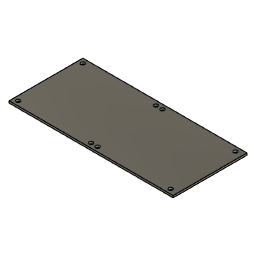
Color Clock asssebly v13 (Autodesk Fusion 360 archive; units mm, degrees)
design "prototype board test"
Autodesk Fusion 360 part; units mm, degrees
sketch "Sketch1" plane through (0, 0, 0) normal (0, 0, 1) x (1, 0, 0)
  line L0 (0, 0) -> (50, 0)
  line L1 (50, 0) -> (50, 45)
  line L2 (50, 45) -> (0, 45)
  line L3 (0, 45) -> (0, 0)
  line L4 (47.25, 42.25) -> (2.75, 42.25)
  line L5 (2.75, 42.25) -> (2.75, 2.75)
  line L6 (2.75, 2.75) -> (47.25, 2.75)
  line L7 (47.25, 2.75) -> (47.25, 42.25)
  line L8 (47.25, 42.25) -> (2.75, 2.75) construction
  line L9 (2.75, 42.25) -> (47.25, 2.75) construction
  line L10 (50, 45) -> (0, 0) construction
  circle A0 centre (2.75, 42.25) radius 1.2
  circle A1 centre (2.75, 2.75) radius 1.2
  circle A2 centre (47.25, 42.25) radius 1.2
  circle A3 centre (47.25, 2.75) radius 1.2
  line L11 (95.75, 2.75) -> (95.75, 42.25)
  line L12 (51.25, 2.75) -> (95.75, 2.75)
  line L13 (98.5, 45) -> (48.5, 0) construction
  line L14 (51.25, 42.25) -> (95.75, 2.75) construction
  line L15 (95.75, 42.25) -> (51.25, 2.75) construction
  circle A4 centre (51.25, 42.25) radius 1.2
  circle A5 centre (51.25, 2.75) radius 1.2
  line L16 (95.75, 42.25) -> (51.25, 42.25)
  circle A6 centre (95.75, 42.25) radius 1.2
  circle A7 centre (95.75, 2.75) radius 1.2
  line L17 (51.25, 42.25) -> (51.25, 2.75)
  line L18 (50, 45) -> (100, 45)
  line L19 (100, 45) -> (100, 0)
  line L20 (100, 0) -> (50, 0)
  line L21 (50, 0) -> (50, 45)
  point P0 (25, 22.5)
  point P1 (73.5, 22.5)
  dimension "d1" = 50
  dimension "d2" = 44.5
  dimension "d3" = 39.5
  dimension "d4" = 2.4
  dimension "d5" = 2.4
  dimension "d6" = 2.4
  dimension "d7" = 2.4
  dimension "d12" = 45
  dimension "d14" = 44.5
  dimension "d15" = 39.5
  dimension "d16" = 2.4
  dimension "d17" = 2.4
  dimension "d18" = 2.4
  dimension "d19" = 2.4
  dimension "d22" = 4
  dimension "d23" = 100
  dimension "d24" = 45
  dimension "d25" = 4.25
  constraint horizontal L0
  constraint vertical L1
  constraint horizontal L2
  constraint vertical L3
  constraint coincident L0.start L3.end
  constraint horizontal L4
  constraint perpendicular L4 L5
  constraint parallel L4 L6
  constraint parallel L5 L7
  constraint coincident L8 P0
  constraint coincident L9 P0
  constraint midpoint P0 L10
  constraint coincident L4.end L5.start
  constraint coincident L5.end L6.start
  constraint coincident L4.start L7.end
  constraint coincident L6.end L7.start
  constraint horizontal L16
  constraint perpendicular L16 L17
  constraint parallel L12 L16
  constraint parallel L11 L17
  constraint coincident P1 L15
  constraint coincident P1 L14
  constraint midpoint P1 L13
  constraint coincident L14.start A4.centre
  constraint coincident L12.start L15.end
  constraint coincident L11.end L15.start
  constraint coincident L11.start L12.end
  constraint horizontal L18
  constraint vertical L19
  constraint horizontal L20
  constraint vertical L21
  measures "d1" distance of L0.start L0.end
  measures "d2" distance of L5.end L6.end
  measures "d3" distance of L4.end L5.end
  measures "d4" diameter of A0
  measures "d5" diameter of A1
  measures "d6" diameter of A2
  measures "d7" diameter of A3
  measures "d12" distance of L0 L2
  measures "d14" distance of L11.start L12.start
  measures "d15" distance of L14.start L12.start
  measures "d16" diameter of A4
  measures "d17" diameter of A5
  measures "d18" diameter of A6
  measures "d19" diameter of A7
  measures "d22" distance of L4.start L14.start
  measures "d23" distance of L3 L19
  measures "d24" distance of L18 L20
  measures "d25" distance of L11 L19
extrude "Extrude1" add sketch "Sketch1" along normal blind 1.2 contours L0 L1 L2 L3 L21 | L4 L5 L6 L7 A0 A1 A2 A3
extrude "Extrude3" add sketch "Sketch1" along normal blind 1.2 contours L1 L18 L19 L20 L21 | L11 L12 A4 A5 L16 A6 A7 L17

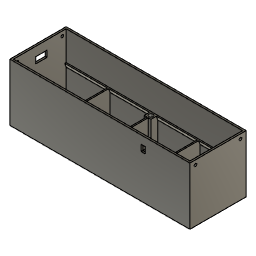
design "Shell"
Autodesk Fusion 360 part; units mm, degrees
derive "DerivedContext1" from "Color Clock asssebly v3"
derive "DerivedContext2" from "Color Clock asssebly v10"
sketch "Sketch1" plane through (0, 0, 0) normal (0, 0, 1) x (1, 0, 0)
  line L0 (0, 0) -> (160, 0)
  line L1 (160, 0) -> (160, 40)
  line L2 (160, 40) -> (0, 40)
  line L3 (0, 40) -> (0, 0)
  dimension "d1" = 160
  dimension "d2" = 40
  constraint horizontal L0
  constraint vertical L1
  constraint horizontal L2
  constraint vertical L3
  constraint coincident L0.start L3.end
  measures "d1" distance of L0.start L0.end
  measures "d2" distance of L0.start L2.end
extrude "Extrude1" add sketch "Sketch1" along normal blind 3 makes body 1
sketch "Sketch2" plane through (0, 0, 3) normal (0, 0, 1) x (-1, 0, 0)
  line L0 (0, -40) -> (0, 0)
  line L1 (0, 0) -> (-160, 0)
  line L2 (-160, 0) -> (-160, -40)
  line L3 (-160, -40) -> (0, -40)
  line L4 (-1.6, -1.6) -> (-158.4, -1.6)
  line L5 (-158.4, -1.6) -> (-158.4, -38.4)
  line L6 (-158.4, -38.4) -> (-1.6, -38.4)
  line L7 (-1.6, -38.4) -> (-1.6, -1.6)
  dimension "d5" = -1.6
extrude "Extrude2" add sketch "Sketch2" along normal blind 50 bodies 1
extrude "Extrude3" cut 1 faces at (53.8667, 39.4667, 53) along direction (0, 0, -1) blind 3 on bodies 1 bodies 1
sketch "Sketch3" plane through (0, 0, 0) normal (0, 0, -1) x (1, 0, 0)
  line L0 (0, 0) -> (0, -40)
  line L1 (0, -40) -> (160, -40)
  line L2 (160, -40) -> (160, 0)
  line L3 (160, 0) -> (0, 0)
  line L4 (40, 0) -> (40, -40)
  line L5 (80, 0) -> (80, -40)
  line L6 (120, 0) -> (120, -40)
  line L7 (39.6, 0) -> (39.6, -40)
  line L8 (40.4, 0) -> (40.4, -40)
  line L9 (79.6, 0) -> (79.6, -40)
  line L10 (80.4, 0) -> (80.4, -40)
  line L11 (119.6, 0) -> (119.6, -40)
  line L12 (120.4, 0) -> (120.4, -40)
  dimension "d10" = 40
  dimension "d11" = 40
  dimension "d12" = 40
  dimension "d14" = 0.4
  dimension "d15" = -0.4
  dimension "d16" = 0.4
  dimension "d17" = -0.4
  dimension "d18" = 0.4
  dimension "d19" = -0.4
  constraint coincident L3 L4.start
  constraint perpendicular L3 L4
  constraint coincident L3 L5.start
  constraint coincident L1 L5.end
  constraint perpendicular L1 L5
  constraint coincident L3 L6.start
  constraint coincident L1 L6.end
  constraint perpendicular L1 L6
  measures "d10" distance of L0 L4
  measures "d11" distance of L4 L5
  measures "d12" distance of L5 L6
extrude "Extrude4" add sketch "Sketch3" against normal blind 25 contours L1 L3 L4 L7 | L1 L3 L4 L8 | L1 L3 L5 L9 | L1 L3 L5 L10 | L1 L3 L6 L11 | L1 L3 L6 L12 bodies 1
sketch "Sketch4" plane through (0, 0, 25) normal (0, 0, 1) x (-1, 0, 0)
  line L0 (-80.4, -38.4) -> (-79.6, -38.4)
  line L1 (-79.6, -38.4) -> (-79.6, -1.6)
  line L2 (-79.6, -1.6) -> (-80.4, -1.6)
  line L3 (-80.4, -1.6) -> (-80.4, -38.4)
  circle A0 centre (-80, -35.4) radius 1.9
  line L4 (-77, -38.4) -> (-83, -38.4)
  line L5 (-83, -38.4) -> (-83, -32.4)
  line L6 (-83, -32.4) -> (-77, -32.4)
  line L7 (-77, -32.4) -> (-77, -38.4)
  line L8 (-158.4, -38.4) -> (-1.6, -38.4)
  circle A1 centre (-80, -4.6) radius 1.9
  line L9 (-77, -7.6) -> (-83, -7.6)
  line L10 (-83, -7.6) -> (-83, -1.6)
  line L11 (-83, -1.6) -> (-77, -1.6)
  line L12 (-77, -1.6) -> (-77, -7.6)
  dimension "d22" = 3.8
  dimension "d23" = 3
  dimension "d24" = 3
  dimension "d25" = 3
  dimension "d26" = 3
  dimension "d27" = 3.8
  dimension "d28" = 3
  dimension "d29" = 6
  dimension "d30" = 3
  dimension "d31" = 6
  constraint horizontal L4
  constraint vertical L5
  constraint horizontal L6
  constraint vertical L7
  constraint collinear L4 L8
  constraint midpoint L0 L4
  constraint horizontal L9
  constraint vertical L10
  constraint horizontal L11
  constraint vertical L12
  constraint midpoint L2 L11
  measures "d22" diameter of A0
  measures "d23" distance of A0.centre L5
  measures "d24" distance of A0.centre L7
  measures "d25" distance of A0.centre L6
  measures "d26" distance of A0.centre L4
  measures "d27" diameter of A1
  measures "d28" distance of A1.centre L9
  measures "d29" distance of L9 L11
  measures "d30" distance of A1.centre L10
  measures "d31" distance of L10 L12
extrude "Extrude5" add sketch "Sketch4" against normal blind 22 contours L3 A0 L4 L5 L6 L8 | L1 A0 L4 L6 L7 L8 | L3 A0 | L1 A0 | L3 A1 L9 L10 L11 | L1 A1 L9 L11 L12 | L3 A1 | L1 A1 bodies 1
hole "Hole1" at (80, 35.4, 25) at (80, 4.6, 25) direction (0, 0, -1) diameter 3.5 depth 8 tip angle 180 countersink diameter 3.8 countersink angle 6 bodies 1
sketch "Sketch5" plane through (0, 0, 25) normal (0, 0, 1) x (-1, 0, 0)
  line L0 (-80, -4.5) -> (-80, -35.5)
  constraint vertical L0
sketch "Sketch6" plane through (0, 0, 0) normal (-1, 0, 0) x (0, -1, 0)
  line L0 (0, 50) -> (-40, 50)
  line L1 (-40, 50) -> (-40, 0)
  line L2 (-40, 0) -> (0, 0)
  line L3 (0, 0) -> (0, 50)
  line L4 (-35, 46) -> (-5, 46) construction
  constraint parallel L0 L4
hole "Hole2" at (0, 35, 46) at (0, 5, 46) direction (1, 0, 0) diameter 2.25 depth 196 tip angle 180 bodies 1
sketch "Sketch7" plane through (0, 40, 0) normal (0, 1, 0) x (-1, 0, 0)
  line L0 (-160, 0) -> (0, 0)
  line L1 (0, 0) -> (0, 50)
  line L2 (0, 50) -> (-160, 50)
  line L3 (-160, 50) -> (-160, 0)
  line L4 (-17.4, 37.15) -> (-22.6, 37.15)
  line L5 (-22.6, 37.15) -> (-22.6, 32.85)
  line L6 (-22.6, 32.85) -> (-17.4, 32.85)
  line L7 (-17.4, 32.85) -> (-17.4, 37.15)
  line L8 (-17.4, 37.15) -> (-22.6, 32.85) construction
  line L9 (-22.6, 37.15) -> (-17.4, 32.85) construction
  line L10 (-80, 25) -> (-80, 50) construction
  line L11 (0, 50) -> (0, 0)
  line L12 (-23.6, 31.85) -> (-16.4, 31.85)
  line L13 (-16.4, 31.85) -> (-16.4, 38.15)
  line L14 (-16.4, 38.15) -> (-23.6, 38.15)
  line L15 (-23.6, 38.15) -> (-23.6, 31.85)
  line L16 (-22.6, 37.15) -> (-22.6, 38.15)
  line L17 (-17.4, 37.15) -> (-17.4, 38.15)
  point P0 (-20, 35)
  dimension "d42" = 5.2
  dimension "d43" = 4.3
  dimension "d44" = 15
  dimension "d45" = 20
  dimension "d48" = 1
  constraint horizontal L4
  constraint perpendicular L4 L5
  constraint parallel L4 L6
  constraint parallel L5 L7
  constraint coincident L8 P0
  constraint coincident L9 P0
  constraint midpoint L2 L10.end
  constraint coincident L14 L16.end
  constraint perpendicular L14 L16
  constraint coincident L14 L17.end
  constraint perpendicular L14 L17
  measures "d42" distance of L5.end L6.end
  measures "d43" distance of L4.end L5.end
  measures "d44" distance of L2 P0
  measures "d45" distance of P0 L11
extrude "Extrude6" cut sketch "Sketch7" against normal blind 9 contours L4 L5 L6 L7 bodies 1
extrude "Extrude7" add sketch "Sketch7" against normal blind 2.5 contours L5 L6 L7 L12 L13 L14 L15 L16 L17 bodies 1
fillet "Fillet1" radius 1 3 edges at (20, 37.5, 31.85) (16.4, 37.5, 35) (23.6, 37.5, 35) on bodies 1
ref_plane "WorkPlane1" through (80, 20, 26.5) normal (0, 1, 0) x (-1, 0, 0)
split "Split1" by plane through (80, 20, 26.5) normal (0, 1, 0) bodies 1 makes body 2 at (114.2, 40, 27.6167)
move_body "Move1" bodies 1 to x (1, 0, 0) y (0, 1, 0) z (0, 0, 1) at (0, -10, 0)
extrude "Extrude8" add 1 faces at (66.5333, 10, 1) along direction (0, 1, 0) blind 10 on bodies 1 bodies 1 2
extrude "Extrude9" add 1 faces at (19.1333, 39.4667, 37.15) along direction (0, 0, -1) blind 5 on bodies 1 bodies 1
extrude "Extrude10" cut 1 faces at (20.8667, 38.1, 32.85) along direction (0, 0, -1) blind 4 on bodies 1 bodies 1
extrude "Extrude11" cut 1 faces at (22.6, 38.1, 34.285) along direction (-1, 0, 0) blind 8 and the other way blind 4 on bodies 1 bodies 1
sketch "Sketch8" plane through (0, 38.4, 0) normal (0, -1, 0) x (1, 0, 0)
  line L0 (77, 25) -> (83, 25)
  line L1 (83, 25) -> (83, 3)
  line L2 (83, 3) -> (119.6, 3)
  line L3 (119.6, 3) -> (119.6, 25)
  line L4 (119.6, 25) -> (120.4, 25)
  line L5 (120.4, 25) -> (120.4, 3)
  line L6 (120.4, 3) -> (158.4, 3)
  line L7 (158.4, 3) -> (158.4, 50)
  line L8 (158.4, 50) -> (1.6, 50)
  line L9 (1.6, 50) -> (1.6, 3)
  line L10 (1.6, 3) -> (39.6, 3)
  line L11 (39.6, 3) -> (39.6, 25)
  line L12 (39.6, 25) -> (40.4, 25)
  line L13 (40.4, 25) -> (40.4, 3)
  line L14 (40.4, 3) -> (77, 3)
  line L15 (77, 3) -> (77, 25)
  line L16 (108.5, 43) -> (118.5, 43) construction
  line L17 (118.5, 25) -> (118.5, 41) construction
  line L18 (120.3, 43.75) -> (116.7, 43.75)
  line L19 (116.7, 43.75) -> (116.7, 38.25)
  line L20 (116.7, 38.25) -> (120.3, 38.25)
  line L21 (120.3, 38.25) -> (120.3, 43.75)
  line L22 (120.3, 43.75) -> (116.7, 38.25) construction
  line L23 (116.7, 43.75) -> (120.3, 38.25) construction
  point P0 (118.5, 41)
  dimension "d63" = 10
  dimension "d64" = 3.6
  dimension "d65" = 5.5
  constraint horizontal L16
  constraint horizontal L18
  constraint perpendicular L18 L19
  constraint parallel L18 L20
  constraint parallel L19 L21
  constraint coincident L22 P0
  constraint coincident L23 P0
  constraint coincident P0 L17.end
  measures "d63" distance of L16.start L16.end
  measures "d64" distance of L19.end L20.end
  measures "d65" distance of L18.end L19.end
extrude "Extrude12" cut sketch "Sketch8" against normal blind 4 contours L18 L19 L20 L21 bodies 1
sketch "Sketch9" plane through (0, 38.4, 0) normal (0, -1, 0) x (1, 0, 0)
  line L0 (116.7, 43.75) -> (120.3, 43.75)
  line L1 (120.3, 43.75) -> (120.3, 38.25)
  line L2 (120.3, 38.25) -> (116.7, 38.25)
  line L3 (116.7, 38.25) -> (116.7, 43.75)
  line L4 (77, 25) -> (83, 25)
  line L5 (83, 25) -> (83, 3)
  line L6 (83, 3) -> (119.6, 3)
  line L7 (119.6, 3) -> (119.6, 25)
  line L8 (119.6, 25) -> (120.4, 25)
  line L9 (120.4, 25) -> (120.4, 3)
  line L10 (120.4, 3) -> (158.4, 3)
  line L11 (158.4, 3) -> (158.4, 50)
  line L12 (158.4, 50) -> (1.6, 50)
  line L13 (1.6, 50) -> (1.6, 3)
  line L14 (1.6, 3) -> (39.6, 3)
  line L15 (39.6, 3) -> (39.6, 25)
  line L16 (39.6, 25) -> (40.4, 25)
  line L17 (40.4, 25) -> (40.4, 3)
  line L18 (40.4, 3) -> (77, 3)
  line L19 (77, 3) -> (77, 25)
  line L20 (116.3, 43.95) -> (116.3, 38.05)
  line L21 (116.3, 38.05) -> (120.7, 38.05)
  line L22 (120.7, 38.05) -> (120.7, 43.95)
  line L23 (120.7, 43.95) -> (116.3, 43.95)
  line L24 (115.5, 44.5062) -> (115.5, 37.25)
  line L25 (115.5, 37.25) -> (121.5, 37.25)
  line L26 (121.5, 37.25) -> (121.5, 44)
  line L27 (115.5, 43.95) -> (121.5, 43.95)
  dimension "d68" = 0.4
  dimension "d69" = 0.4
  dimension "d70" = 0.2
  dimension "d72" = 0.2
  dimension "d73" = 0.8
  dimension "d74" = 0.8
  dimension "d75" = 0.8
  dimension "d76" = 0.2
  constraint perpendicular L12 L20
  constraint perpendicular L20 L21
  constraint perpendicular L12 L22
  constraint parallel L0 L23
  constraint perpendicular L22 L25
  constraint perpendicular L25 L26
  constraint parallel L20 L24
  constraint coincident L24 L27.start
  constraint coincident L26 L27.end
  constraint perpendicular L26 L27
  measures "d68" distance of L3 L20
  measures "d69" distance of L1 L22
  measures "d70" distance of L2 L21
  measures "d72" distance of L0 L23
  measures "d73" distance of L20 L24
  measures "d74" distance of L22 L26
  measures "d75" distance of L21 L25
  measures "d76" distance of L0 L27
extrude "Extrude13" add sketch "Sketch9" along normal blind 3.4 contours L20 L21 L22 L24 L25 L26 L27 bodies 1
sketch "Sketch10" plane through (0, 0, 38.05) normal (0, 0, 1) x (-1, 0, 0)
  line L0 (-120.7, -38.4) -> (-116.3, -38.4)
  line L1 (-116.3, -38.4) -> (-116.3, -35)
  line L2 (-116.3, -35) -> (-120.7, -35)
  line L3 (-120.7, -35) -> (-120.7, -38.4)
  line L4 (-116.3, -35) -> (-120.7, -35)
  line L5 (-120.7, -35) -> (-120.7, -35.8)
  line L6 (-120.7, -35.8) -> (-116.3, -35.8)
  line L7 (-116.3, -35.8) -> (-116.3, -35)
  line L8 (-117.7, -35.8) -> (-119.3, -35.8)
  line L9 (-119.3, -35.8) -> (-119.3, -35)
  line L10 (-119.3, -35) -> (-117.7, -35)
  line L11 (-117.7, -35) -> (-117.7, -35.8)
  dimension "d79" = 4.4
  dimension "d80" = 0.8
  dimension "d81" = 1.6
  dimension "d82" = 1.4
  constraint horizontal L4
  constraint vertical L5
  constraint horizontal L6
  constraint vertical L7
  constraint coincident L1.end L2.start
  constraint horizontal L8
  constraint vertical L9
  constraint horizontal L10
  constraint vertical L11
  constraint coincident L6 L8.start
  measures "d79" distance of L1.end L2.end
  measures "d80" distance of L1.end L6.end
  measures "d81" distance of L8.start L8.end
  measures "d82" distance of L7 L11
extrude "Extrude14" add sketch "Sketch10" along normal blind 5.9 contours L2 L3 L4 L5 L6 L9 | L1 L2 L4 L6 L7 L11 bodies 1
extrude "Extrude15" add sketch "Sketch10" along normal blind 1 contours L2 L4 L6 L8 L9 L10 L11 bodies 1
sketch "Sketch11" plane through (115.5, 0, 0) normal (-1, 0, 0) x (0, -1, 0)
  line L0 (-38.4, 43.95) -> (-38.4, 37.25)
  line L1 (-38.4, 37.25) -> (-35, 37.25)
  line L2 (-35, 37.25) -> (-35, 43.95)
  line L3 (-35, 43.95) -> (-38.4, 43.95)
  line L4 (-35, 37.25) -> (-38.4, 33.85)
  line L5 (-35, 37.25) -> (-30.1917, 37.25) construction
  line L6 (-38.4, 33.85) -> (-38.4, 37.25)
  dimension "d87" = 135
  constraint horizontal L5
  constraint coincident L1.end L2.start
  constraint coincident L0.end L1.start
  constraint perpendicular L1 L6
  measures "d87" angle of L4 L5
extrude "Extrude16" add sketch "Sketch11" against normal blind 6 contours L1 L4 L6 bodies 1
sketch "Sketch12" plane through (1.6, 0, 0) normal (1, 0, 0) x (0, 1, 0)
  circle A0 centre (35, 46) radius 1.125
  line L0 (38.4, 50) -> (-8.4, 50)
  line L1 (-8.4, 50) -> (-8.4, 3)
  line L2 (-8.4, 3) -> (38.4, 3)
  line L3 (38.4, 3) -> (38.4, 50)
  circle A1 centre (-5, 46) radius 1.125
  line L4 (38.4, 37) -> (-8.4, 37)
  line L5 (-8.4, 43.5) -> (38.4, 43.5)
  line L6 (10.9, 43.5) -> (10.9, 37)
  line L7 (21.9, 43.5) -> (21.9, 37)
  point P0 (38.4, 25)
  dimension "d90" = 46.8
  dimension "d91" = 12
  dimension "d92" = 18.5
  dimension "d93" = 11
  dimension "d94" = 16.5
  constraint horizontal L4
  constraint coincident L3 L4.start
  constraint coincident L1 L4.end
  constraint coincident L1 L5.start
  constraint perpendicular L3 L5
  constraint coincident L5 L6.start
  constraint coincident L4 L6.end
  constraint perpendicular L4 L6
  constraint coincident L5 L7.start
  constraint coincident L4 L7.end
  constraint perpendicular L4 L7
  measures "d90" distance of L5.start L5.end
  measures "d91" distance of L4.start P0
  measures "d92" distance of L5.end P0
  measures "d93" distance of L6 L7
  measures "d94" distance of L3 L7
extrude "Extrude17" cut sketch "Sketch12" against normal blind 14 contours L4 L5 L6 L7 bodies 1
extrude "Extrude18" add 1 faces at (39.6, 7.2, 17.6667) along direction (-1, 0, 0) blind 0.2 on bodies 1 bodies 1
extrude "Extrude19" add 1 faces at (40.4, 7.2, 17.6667) along direction (1, 0, 0) blind 0.2 on bodies 1 bodies 1
extrude "Extrude20" add 1 faces at (79.6, 9.2, 10.3333) along direction (-1, 0, 0) blind 0.2 on bodies 1 bodies 1
extrude "Extrude21" add 1 faces at (80.4, 9.2, 10.3333) along direction (1, 0, 0) blind 0.2 on bodies 1 bodies 1
extrude "Extrude22" add 1 faces at (120.4, 7.2, 17.6667) along direction (1, 0, 0) blind 0.2 on bodies 1 bodies 1
extrude "Extrude23" add 1 faces at (119.6, 7.2, 17.6667) along direction (-1, 0, 0) blind 0.2 on bodies 1 bodies 1
extrude "Extrude24" cut sketch "Sketch9" along normal blind 35 from surface at 20 contours L0 L1 L2 L3 bodies 1
sketch "Sketch13" plane through (0, -8.4, 0) normal (0, 1, 0) x (-1, 0, 0)
  line L0 (-116.7, 43.75) -> (-116.7, 38.25)
  line L1 (-116.7, 38.25) -> (-120.3, 38.25)
  line L2 (-120.3, 38.25) -> (-120.3, 43.75)
  line L3 (-120.3, 43.75) -> (-116.7, 43.75)
  line L4 (-120.6, 25) -> (-119.4, 25)
  line L5 (-119.4, 25) -> (-119.4, 3)
  line L6 (-119.4, 3) -> (-83, 3)
  line L7 (-83, 3) -> (-83, 25)
  line L8 (-83, 25) -> (-77, 25)
  line L9 (-77, 25) -> (-77, 3)
  line L10 (-77, 3) -> (-40.6, 3)
  line L11 (-40.6, 3) -> (-40.6, 25)
  line L12 (-40.6, 25) -> (-39.4, 25)
  line L13 (-39.4, 25) -> (-39.4, 3)
  line L14 (-39.4, 3) -> (-1.6, 3)
  line L15 (-1.6, 3) -> (-1.6, 50)
  line L16 (-1.6, 50) -> (-158.4, 50)
  line L17 (-158.4, 50) -> (-158.4, 3)
  line L18 (-158.4, 3) -> (-120.6, 3)
  line L19 (-120.6, 3) -> (-120.6, 25)
  line L20 (-120.7, 43.95) -> (-113.4412, 43.95)
  line L21 (-120.7, 43.95) -> (-120.7, 38.05)
  line L22 (-120.7, 38.05) -> (-116.3, 38.05)
  line L23 (-116.3, 38.05) -> (-116.3, 44.3)
  line L24 (-121.5, 44.5) -> (-121.5, 37.25)
  line L25 (-121.5, 37.25) -> (-115.5, 37.25)
  line L26 (-115.5, 37.25) -> (-115.5, 44.5)
  line L27 (-121.5, 43.95) -> (-115.5, 43.95)
  dimension "d112" = 0.4
  dimension "d113" = 0.4
  dimension "d114" = 0.2
  dimension "d115" = 0.2
  dimension "d116" = 0.8
  dimension "d117" = 0.8
  dimension "d118" = 0.8
  dimension "d119" = 0.2
  constraint perpendicular L2 L20
  constraint perpendicular L20 L21
  constraint perpendicular L21 L22
  constraint perpendicular L22 L23
  constraint vertical L24
  constraint perpendicular L24 L25
  constraint perpendicular L20 L26
  constraint coincident L24 L27.start
  constraint coincident L26 L27.end
  constraint perpendicular L26 L27
  measures "d112" distance of L2 L21
  measures "d113" distance of L0 L23
  measures "d114" distance of L1 L22
  measures "d115" distance of L3 L20
  measures "d116" distance of L21 L24
  measures "d117" distance of L22 L25
  measures "d118" distance of L23 L26
  measures "d119" distance of L3 L27
extrude "Extrude25" add sketch "Sketch13" along normal blind 3.4 contours L20 L21 L22 L23 L24 L25 L26 L27 bodies 1
sketch "Sketch14" plane through (0, 0, 38.05) normal (0, 0, 1) x (-1, 0, 0)
  line L0 (-116.3, 8.4) -> (-120.7, 8.4)
  line L1 (-120.7, 8.4) -> (-120.7, 5)
  line L2 (-120.7, 5) -> (-116.3, 5)
  line L3 (-116.3, 5) -> (-116.3, 8.4)
  line L4 (-116.3, 5.8) -> (-120.7, 5.8)
  line L5 (-117.7, 5) -> (-117.7, 5.8)
  line L6 (-119.3, 5) -> (-119.3, 5.8)
  dimension "d122" = 0.8
  dimension "d123" = 1.6
  dimension "d124" = 1.4
  constraint coincident L3 L4.start
  constraint coincident L1 L4.end
  constraint perpendicular L1 L4
  constraint coincident L2 L5.start
  constraint coincident L4 L5.end
  constraint perpendicular L4 L5
  constraint coincident L2 L6.start
  constraint coincident L4 L6.end
  constraint perpendicular L4 L6
  measures "d122" distance of L2 L4
  measures "d123" distance of L5 L6
  measures "d124" distance of L3 L5
extrude "Extrude26" add sketch "Sketch14" along normal blind 5.9 contours L2 L3 L4 L5 | L1 L2 L4 L6 bodies 1
extrude "Extrude27" add sketch "Sketch14" along normal blind 1 contours L2 L4 L5 L6 bodies 1
sketch "Sketch15" plane through (121.5, 0, 0) normal (1, 0, 0) x (0, 1, 0)
  line L0 (-8.4, 43.95) -> (-8.4, 37.25)
  line L1 (-8.4, 37.25) -> (-5, 37.25)
  line L2 (-5, 37.25) -> (-5, 43.95)
  line L3 (-5, 43.95) -> (-8.4, 43.95)
  line L4 (-5, 37.25) -> (-8.8054, 33.4446)
  line L5 (-5, 37.25) -> (-10.3817, 37.25) construction
  line L6 (-8.8054, 33.4446) -> (-8.8054, 37.25)
  line L7 (-5, 37.25) -> (-8.8054, 37.25)
  dimension "d129" = 45
  constraint horizontal L5
  constraint coincident L1.end L2.start
  constraint coincident L5 L6.end
  constraint perpendicular L5 L6
  measures "d129" angle of L4 L5
extrude "Extrude28" add sketch "Sketch15" against normal blind 6 contours L1 L4 L6 L7 bodies 1
extrude "Extrude29" cut 1 faces at (121.5, 37.2667, 38.35) along direction (-1, 0, 0) blind 12 on bodies 1 bodies 1
extrude "Extrude30" add 1 faces at (117.9, 38.9333, 38.25) along direction (0, 0, 1) blind 6 on bodies 1 bodies 1
extrude "Extrude31" cut 1 faces at (1.0667, 14.5667, 43.5) along direction (0, 0, 1) blind 1.5 on bodies 1 bodies 1
extrude "Extrude32" add 1 faces at (1.0667, 18.2333, 37) along direction (0, 0, 1) blind 2 on bodies 1 bodies 1
extrude "Extrude33" add 1 faces at (1.0667, 10.9, 43) along direction (0, 1, 0) blind 0.5 on bodies 1 bodies 1
extrude "Extrude34" add 1 faces at (1.0667, 21.9, 43) along direction (0, -1, 0) blind 0.5 on bodies 1 bodies 1
split "Split2" by plane through (80, 15, 44) normal (0, 0, 1) bodies 1 makes body 3 at (106.6667, 40, 46)
move_body "Move2" bodies 3 to x (1, 0, 0) y (0, 1, 0) z (0, 0, 1) at (0, 0, 1)
extrude "Extrude35" add 1 faces at (53.8667, 39.4667, 44) along direction (0, 0, 1) blind 1 on bodies 1 bodies 1 3
extrude "Extrude36" add 1 faces at (1.0667, 14.7333, 46) along direction (0, 0, -1) blind 1 on bodies 1 bodies 1
sketch "Sketch16" plane through (160, 0, 0) normal (1, 0, 0) x (0, 1, 0)
  circle A0 centre (-5, 47) radius 1.125
  circle A1 centre (35, 47) radius 1.125
  line L0 (-10, 51) -> (-10, 0)
  line L1 (-10, 0) -> (40, 0)
  line L2 (40, 0) -> (40, 51)
  line L3 (40, 51) -> (-10, 51)
  circle A2 centre (-5, 47) radius 1.1875
  circle A3 centre (35, 47) radius 1.1875
  dimension "d148" = 2.375
  dimension "d149" = 2.375
  constraint concentric A0 A2
  constraint concentric A1 A3
  measures "d148" diameter of A2
  measures "d149" diameter of A3
extrude "Extrude37" cut sketch "Sketch16" against normal blind 180 contours A0 | A1 | A2 | A3 bodies 1
extrude "Extrude38" add 1 faces at (1.0667, 14.7333, 45) along direction (0, 0, -1) blind 2 on bodies 1 bodies 1
extrude "Extrude39" cut 1 faces at (1.0667, 18.0667, 39) along direction (0, 0, -1) blind 1.5 on bodies 1 bodies 1
sketch "Sketch17" plane through (0, 38.4, 0) normal (0, -1, 0) x (1, 0, 0)
  line L0 (9, 25) -> (14, 25)
  line L1 (14, 25) -> (14, 24)
  line L2 (14, 24) -> (9, 24)
  line L3 (9, 24) -> (9, 25)
  constraint horizontal L0
  constraint vertical L1
  constraint horizontal L2
  constraint vertical L3
extrude "Extrude40" add sketch "Sketch17" along normal blind 46.8 bodies 1
sketch "Sketch18" plane through (14, 0, 0) normal (1, 0, 0) x (0, 1, 0)
  line L0 (38.4, 24) -> (38.4, 25)
  line L1 (38.4, 25) -> (-8.4, 25)
  line L2 (-8.4, 25) -> (-8.4, 24)
  line L3 (-8.4, 24) -> (38.4, 24)
  line L4 (38.4, 24) -> (38.4, 21.5)
  line L5 (38.4, 21.5) -> (37.4901, 24)
  line L6 (-8.4, 24) -> (-8.4, 21.5)
  line L7 (-8.4, 21.5) -> (-7.4901, 24)
  line L8 (38.4, 21.5) -> (37.1261, 25)
  line L9 (37.1261, 25) -> (38.4, 25)
  line L10 (38.4, 24) -> (38.4, 21.5)
  line L11 (-8.4, 21.5) -> (-7.1261, 25)
  line L12 (-7.1261, 25) -> (-8.4, 25)
  line L13 (-8.4, 21.5) -> (-8.4, 25)
  dimension "d158" = 20
  dimension "d159" = 20
  constraint coincident L0.start L3.end
  constraint perpendicular L3 L4
  constraint coincident L3 L5.end
  constraint coincident L2.end L3.start
  constraint perpendicular L3 L6
  constraint coincident L3 L7.end
  constraint coincident L1 L8.end
  constraint parallel L5 L8
  constraint coincident L0.end L1.start
  constraint perpendicular L0 L9
  constraint coincident L1 L11.end
  constraint parallel L7 L11
  constraint coincident L1.end L2.start
  measures "d158" angle of L4 L5
  measures "d159" angle of L6 L7
extrude "Extrude41" add sketch "Sketch18" against normal blind 5 contours L3 L4 L5 L8 L10 | L3 L6 L7 L11 L13 bodies 1
extrude "Extrude42" cut sketch "Sketch18" against normal blind 5.5 contours L1 L3 L8 L11 bodies 1
extrude "Extrude43" add 1 faces at (14, -7.9754, 23.8333) along direction (1, 0, 0) blind 5 from surface at 10 on bodies 1 bodies 1
extrude "Extrude44" add 1 faces at (29, -7.9754, 23.8333) along direction (1, 0, 0) blind 5 from surface at 25 on bodies 1 bodies 1
extrude "Extrude45" add 1 faces at (59, -7.9754, 23.8333) along direction (1, 0, 0) blind 5 from surface at 35 on bodies 1 bodies 1
extrude "Extrude46" add 1 faces at (99, -7.9754, 23.8333) along direction (1, 0, 0) blind 5 from surface at 30 on bodies 1 bodies 1
extrude "Extrude47" add 1 faces at (134, -7.9754, 23.8333) along direction (1, 0, 0) blind 15 on bodies 1 bodies 1
extrude "Extrude48" add 1 faces at (99, -7.9754, 23.8333) along direction (1, 0, 0) blind 59.4 on bodies 1 bodies 1
extrude "Extrude49" add 1 faces at (94, -7.9754, 23.8333) along direction (-1, 0, 0) blind 11 on bodies 1 bodies 1
extrude "Extrude50" add 1 faces at (59, -7.9754, 23.8333) along direction (1, 0, 0) blind 18 on bodies 1 bodies 1
extrude "Extrude51" add 1 faces at (54, -7.9754, 23.8333) along direction (-1, 0, 0) blind 52.4 on bodies 1 bodies 1
extrude "Extrude52" add 1 faces at (14, 37.9754, 23.8333) along direction (1, 0, 0) blind 63.5 on bodies 1 bodies 1
extrude "Extrude53" add 1 faces at (9, 38.0967, 23.5) along direction (-1, 0, 0) blind 4 from surface at -100 on bodies 1 bodies 1
extrude "Extrude54" add 1 faces at (105, 38.0967, 23.5) along direction (-1, 0, 0) blind 22 on bodies 1 bodies 1
extrude "Extrude55" add 1 faces at (109, 38.0967, 23.5) along direction (1, 0, 0) blind 49.4 on bodies 1 bodies 1
extrude "Extrude56" add 1 faces at (9, 38.0967, 23.5) along direction (-1, 0, 0) blind 7.4 on bodies 1 bodies 1
